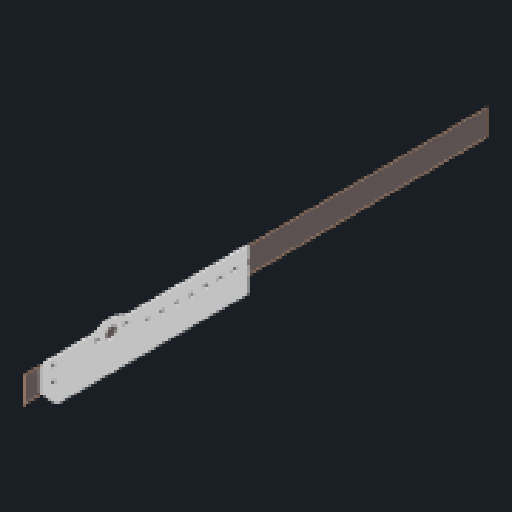
# Autodesk Inventor part: Part1
Saved by Autodesk Inventor 2026.1 (Build 301233000, 233)
## iProperties
Created: 2025-11-04
Part Number: Part1
Material: Generic
Document SubType Name: Modeling
Designer: jasper
Density: 1 g/cm^3
Appearance: Default
Author: jasper
Autodesk Inventor part; units mm, degrees
ref_plane "YZ Plane" through (0, 0, 0) normal (1, 0, 0) x (0, 1, 0)
ref_plane "XZ Plane" through (0, 0, 0) normal (0, 1, 0) x (-1, 0, 0)
ref_plane "XY Plane" through (0, 0, 0) normal (0, 0, 1) x (1, 0, 0)
ref_plane "Work Plane1" through (15.0988, -72.0521, -0.2464) normal (1, 0, 0) x (0, 1, 0)
sketch "Sketch1" plane through (15.0988, -72.0521, -0.2464) normal (1, 0, 0) x (0, 1, 0)
  circle A0 centre (0, 44.45) radius 2.1844 construction
  circle A1 centre (0, 6.35) radius 2.1844 construction
  circle A2 centre (0, 19.05) radius 2.1844 construction
  circle A3 centre (0, 31.75) radius 2.1844 construction
  line L0 (2.3114, -184.15) -> (10.3188, -184.15) construction
  circle A4 centre (0, 6.35) radius 2.1844 construction
  line L1 (61.7311, 6.35) -> (-93.8561, 6.35)
  line L2 (-24.13, 6.35) -> (-24.13, 172.2574)
  line L3 (-22.1107, 176.9015) -> (-10.7194, 187.5241)
  line L4 (-6.3887, 189.23) -> (6.35, 189.23)
  line L5 (12.7, 182.88) -> (12.7, 5.2631)
  line L6 (12.7, 184.15) -> (12.7, 121.7422) projected
  line L7 (-12.7, 121.7422) -> (-12.7, 184.15) projected
  line L8 (10.3187, 184.15) -> (-10.3187, 184.15) projected
  arc A5 (-6.3887, 189.23) -> (-10.7194, 187.5241) centre (-6.3887, 182.88) ccw
  arc A6 (-22.1107, 176.9015) -> (-24.13, 172.2574) centre (-17.78, 172.2574) ccw
  arc A7 (12.7, 182.88) -> (6.35, 189.23) centre (6.35, 182.88) ccw
  circle A8 centre (6.35, 177.8) radius 2.1844 projected
  circle A9 centre (-6.35, 177.8) radius 2.1844 projected
  circle A10 centre (0, 6.35) radius 2.1844 projected
  circle A11 centre (0, 19.05) radius 2.1844 projected
  circle A12 centre (0, 31.75) radius 2.1844 projected
  circle A13 centre (0, 44.45) radius 2.1844 projected
  circle A14 centre (0, 82.55) radius 2.1844 projected
  circle A15 centre (6.35, 127) radius 2.1844 projected
  circle A16 centre (6.35, 127) radius 4.953
  line L9 (12.7, 144.78) -> (12.7, 134.62) construction
  line L10 (12.7, 134.62) -> (25.4, 127) construction
  line L11 (25.4, 127) -> (12.7, 119.38) construction
  line L12 (12.7, 119.38) -> (12.7, 109.22) construction
  spline S0 degree 4 poles (12.7, 144.78) (12.7, 134.62) (25.4, 127) (12.7, 119.38) (12.7, 109.22) knots 1 1 1 1 1 2 2 2 2 2
  circle A17 centre (6.35, 139.7) radius 2.1844 projected
  circle A18 centre (6.35, 114.3) radius 2.1844 projected
  circle A19 centre (0, 69.85) radius 2.1844 projected
  circle A20 centre (0, 95.25) radius 2.1844 projected
  circle A21 centre (0, 57.15) radius 2.1844 projected
  circle A22 centre (0, 31.75) radius 2.1844 projected
  circle A23 centre (0, 19.05) radius 2.1844 projected
  point P0 (72.0521, 0.2464)
  point P1 (-8.89, 189.23)
  point P2 (12.7, 189.23)
  point P3 (-2.1844, 6.35)
  point P4 (2.1844, 6.35)
  point P5 (12.7, 6.35)
  dimension "d0" = 11.43
  dimension "d1" = 133
  dimension "d2" = 5.08
  dimension "d3" = 21.59
  dimension "d4" = 6.35
  dimension "d5" = 9.906
  dimension "d6" = 7.62
  dimension "d7" = 7.62
  dimension "d8" = 10.16
  dimension "d9" = 10.16
  dimension "d10" = 12.7
  constraints: 10 end point, 7 point on line, 6 point on circle, 6 tangent, 4 centre point, 3 perpendicular, 3 vertical alignment, 2 equal radius, 1 coincident, 1 collinear, 1 horizontal, 1 horizontal alignment, 3 other
  measures "d0" distance between parallel lines of L2 L7
  measures "d1" angle of L2 L3
  measures "d2" distance between parallel lines of L4 L8
  measures "d3" distance of point (-8.89, 189.23) point (12.7, 189.23)
  measures "d4" radius of A5
  measures "d5" diameter of A16
  measures "d6" vertical distance of L9.end L10.end
  measures "d7" vertical distance of L11.end L10.end
  measures "d8" distance of L9.start L9.end
  measures "d9" distance of L11.end L12.end
  measures "d10" horizontal distance of L11.end L10.end
extrude "Extrusion1" add sketch "Sketch1" along normal blind 1.5875 contours L1 A10 L2 A6 L3 A5 L4 A7 L5 | L5 S0
body "Solid1"
